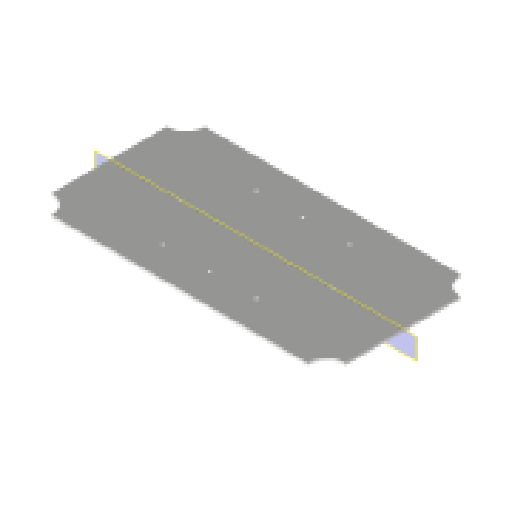
# Autodesk Inventor part: 00_ElectroWallbox_Tpelectric_130x220x140_IP67_Inlet
Saved by Autodesk Inventor 2024.1 (Build 281209000, 209)
## iProperties
Created: 2024-03-15
Part Number: 00_ElectroWallbox_Tpelectric_130x220x140_IP67_Inlet
Material: Generisch
Document SubType Name: Modeling
Designer: diederichbenedict
Density: 1 g/cm^3
Appearance: Vorgabe
Author: diederichbenedict
Autodesk Inventor part; units mm, degrees
ref_plane "YZ Plane" through (0, 0, 0) normal (1, 0, 0) x (0, 1, 0)
ref_plane "XZ Plane" through (0, 0, 0) normal (0, 1, 0) x (-1, 0, 0)
ref_plane "XY Plane" through (0, 0, 0) normal (0, 0, 1) x (1, 0, 0)
sketch "Skizze1" plane through (0, 0, 0) normal (0, 0, 1) x (1, 0, 0)
  line L0 (115, -60) -> (-115, -60)
  line L1 (-115, -60) -> (-115, 60)
  line L2 (-115, 60) -> (115, 60)
  line L3 (115, 60) -> (115, -60)
  line L4 (115, -60) -> (-115, 60) construction
  line L5 (-115, -60) -> (115, 60) construction
  circle A0 centre (-115, 60) radius 15
  circle A1 centre (115, 60) radius 15
  circle A2 centre (115, -60) radius 15
  circle A3 centre (-115, -60) radius 15
  point P0 (0, 0)
  point P1 (-115, -45)
  point P2 (-100, -60)
  point P3 (100, -60)
  point P4 (115, -45)
  point P5 (115, 45)
  point P6 (100, 60)
  point P7 (-100, 60)
  point P8 (-115, 45)
  dimension "d0" = 230
  dimension "d1" = 120
  dimension "d2" = 30
  dimension "d3" = 30
  dimension "d4" = 30
  dimension "d5" = 30
  constraints: 12 end point, 4 centre point, 4 coincident, 2 midpoint, 2 parallel, 1 horizontal, 1 perpendicular
  measures "d0" distance of L1.end L2.end
  measures "d1" distance of L0.end L1.end
  measures "d2" diameter of A0
  measures "d3" diameter of A1
  measures "d4" diameter of A2
  measures "d5" diameter of A3
extrude "Extrusion1" add sketch "Skizze1" along normal blind 2 contours A3 L1 A0 L2 A1 L3 A2 L0
sketch "Skizze2" plane through (0, 0, 2) normal (0, 0, 1) x (1, 0, 0)
  line L0 (36.5, -36.5) -> (-36.5, -36.5)
  line L1 (-36.5, -36.5) -> (-36.5, 36.5)
  line L2 (-36.5, 36.5) -> (36.5, 36.5)
  line L3 (36.5, 36.5) -> (36.5, -36.5)
  line L4 (36.5, -36.5) -> (-36.5, 36.5) construction
  line L5 (-36.5, -36.5) -> (36.5, 36.5) construction
  point P0 (0, 0)
  point P1 (0, 36.5)
  point P2 (0, -36.5)
  point P3 (60, 0)
  point P4 (-60, 0)
  dimension "d8" = 73
  dimension "d9" = 73
  dimension "d25" = 23.5
  dimension "d26" = 23.5
  constraints: 12 end point, 4 coincident, 4 midpoint, 2 parallel, 1 horizontal, 1 perpendicular
  measures "d8" distance of L1.end L2.end
  measures "d9" distance of L0.end L1.end
  measures "d25" horizontal distance of point (-60, 0) L1.end
  measures "d26" horizontal distance of L2.end point (60, 0)
hole "Bohrung1" at (0, 36.5, 2) at (0, -36.5, 2) at (-36.5, -36.5, 2) at (-36.5, 36.5, 2) at (36.5, 36.5, 2) at (36.5, -36.5, 2) at (-60, 0, 2) at (60, 0, 2) direction (0, 0, -1) diameter 2.8 end through all
sketch "Skizze3" plane through (0, 0, 0) normal (0, 0, -1) x (-1, 0, 0)
  circle A0 centre (-36.5, -36.5) radius 1.4 projected
  circle A1 centre (-36.5, 36.5) radius 1.4 projected
  circle A2 centre (36.5, 36.5) radius 1.4 projected
  circle A3 centre (36.5, -36.5) radius 1.4 projected
  circle A4 centre (0, -36.5) radius 1.4 projected
  circle A5 centre (0, 36.5) radius 1.4 projected
  line L0 (100, -60) -> (-100, -60) projected
  arc A6 (115, -45) -> (100, -60) centre (115, -60) ccw projected
  line L1 (115, 45) -> (115, -45) projected
  arc A7 (100, 60) -> (115, 45) centre (115, 60) ccw projected
  line L2 (-100, 60) -> (100, 60) projected
  arc A8 (-115, 45) -> (-100, 60) centre (-115, 60) ccw projected
  line L3 (-115, -45) -> (-115, 45) projected
  arc A9 (-100, -60) -> (-115, -45) centre (-115, -60) ccw projected
  circle A10 centre (36.5, -36.5) radius 5
  circle A11 centre (0, -36.5) radius 5
  circle A12 centre (-36.5, -36.5) radius 5
  circle A13 centre (-36.5, 36.5) radius 5
  circle A14 centre (0, 36.5) radius 5
  circle A15 centre (36.5, 36.5) radius 5
  circle A16 centre (-60, 0) radius 1.4 projected
  circle A17 centre (60, 0) radius 1.4 projected
  circle A18 centre (-36.5, -36.5) radius 1.4 projected
  circle A19 centre (-36.5, 36.5) radius 1.4 projected
  circle A20 centre (36.5, 36.5) radius 1.4 projected
  circle A21 centre (36.5, -36.5) radius 1.4 projected
  circle A22 centre (0, -36.5) radius 1.4 projected
  circle A23 centre (0, 36.5) radius 1.4 projected
  line L4 (100, -60) -> (-100, -60) projected
  arc A24 (115, -45) -> (100, -60) centre (115, -60) ccw projected
  line L5 (115, 45) -> (115, -45) projected
  arc A25 (100, 60) -> (115, 45) centre (115, 60) ccw projected
  line L6 (-100, 60) -> (100, 60) projected
  arc A26 (-115, 45) -> (-100, 60) centre (-115, 60) ccw projected
  line L7 (-115, -45) -> (-115, 45) projected
  arc A27 (-100, -60) -> (-115, -45) centre (-115, -60) ccw projected
  circle A28 centre (60, 0) radius 5
  circle A29 centre (-60, 0) radius 5
  point P0 (0, 0)
  dimension "d17" = 10
  dimension "d18" = 10
  dimension "d19" = 10
  dimension "d20" = 10
  dimension "d21" = 10
  dimension "d22" = 10
  dimension "d27" = 10
  dimension "d28" = 10
  constraints: 8 centre point, 8 coincident
  measures "d17" diameter of A10
  measures "d18" diameter of A11
  measures "d19" diameter of A12
  measures "d20" diameter of A13
  measures "d21" diameter of A14
  measures "d22" diameter of A15
  measures "d27" diameter of A28
  measures "d28" diameter of A29
extrude "Extrusion2" add sketch "Skizze3" along normal blind 13.5 contours A10 | A11 | A12 | A13 | A14 | A15 | A28 | A29
ref_plane "Arbeitsebene1" through (-100, 0, 0) normal (0, 1, 0) x (1, 0, 0)
ref_plane "Arbeitsebene2" through (0, -45, 0) normal (-1, 0, 0) x (0, 0, 1)
